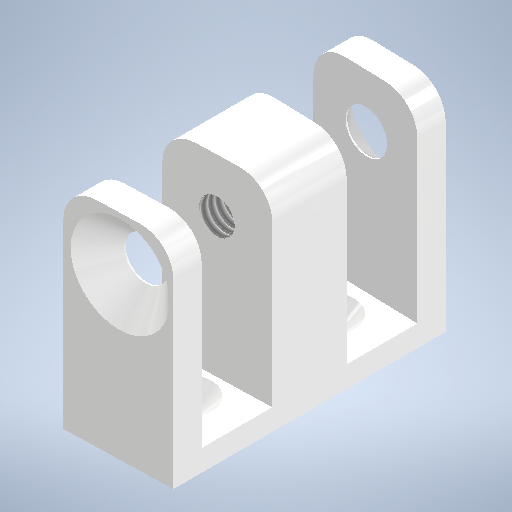
# Autodesk Inventor part: HalterUmlenkrolleDPL
Saved by Autodesk Inventor 2025 (Build 290162010, 162A)
## iProperties
Created: 2024-11-18
Part Number: HalterUmlenkrolleDPL
Material: PC/ABS-Kunststoff, 3DDruck, PLA
Document SubType Name: Modeling
Designer: Admin
Density: 1.1 g/cm^3
Appearance: Glatt - Weiß(2)
Mass: 2.69194 g
Surface Area: 21.9285 cm^2
Volume: 2.44721 cm^3
Author: Admin
Autodesk Inventor part; units mm, degrees
note: some values were not read from the file. Chosen so that the rebuilt part matches the saved one: direction of "Bohrung5"; direction of "Bohrung7".
ref_plane "YZ Plane" through (0, 0, 0) normal (1, 0, 0) x (0, 1, 0)
ref_plane "XZ Plane" through (0, 0, 0) normal (0, 1, 0) x (-1, 0, 0)
ref_plane "XY Plane" through (0, 0, 0) normal (0, 0, 1) x (1, 0, 0)
sketch "Skizze1" plane through (0, 0, 0) normal (0, 0, 1) x (1, 0, 0)
  line L0 (12.8939, 29.9442) -> (2.8939, 30.2214)
  line L1 (2.8939, 30.2214) -> (2.8939, 27.5773)
  line L2 (2.8939, 27.5773) -> (12.8939, 27.3001)
  line L3 (12.8939, 27.3001) -> (12.8939, 29.9442)
  line L4 (12.8939, 7.1427) -> (2.8939, 6.8655)
  line L5 (2.8939, 6.8655) -> (2.8939, 4.2214)
  line L6 (2.8939, 4.2214) -> (12.8939, 4.4985)
  line L7 (12.8939, 4.4985) -> (12.8939, 7.1427)
  line L8 (2.8939, 20.9747) -> (12.8939, 20.6975)
  line L9 (12.8939, 13.7452) -> (2.8939, 13.468)
  line L10 (16.8904, 10.5547) -> (7.8939, 10.3054) construction
  line L11 (16.8904, 23.888) -> (7.8939, 24.1374) construction
  line L12 (16.8904, 10.5547) -> (16.8904, 23.888) construction
  line L13 (2.8939, 20.9747) -> (12.8939, 27.3001) construction
  line L14 (2.8939, 13.468) -> (12.8939, 7.1427) construction
  line L15 (2.8939, 13.468) -> (2.8939, 20.9747)
  line L16 (12.8939, 13.7452) -> (12.8939, 20.6975)
  point P0 (7.8939, 7.0041)
  dimension "d36" = 9
  dimension "d37" = 13.3333
  dimension "d38" = 91.588
  dimension "d39" = 91.588
  dimension "d40" = 10
  dimension "d41" = 6.6
  dimension "d42" = 6.6
  dimension "d43" = 13.8321
  dimension "d58" = 26
  constraints: 34 end point, 6 parallel, 5 collinear, 3 midpoint, 2 vertical, 1 point on line, 1 other
  measures "d36" distance of L10.end L10.start
  measures "d37" distance of L10.start L11.start
  measures "d38" angle of L12 L10
  measures "d39" angle of L12 L11
  measures "d40" distance between parallel lines of L5 L7
  measures "d41" distance between parallel lines of L9 L4
  measures "d42" distance between parallel lines of L2 L8
  measures "d43" distance of L11.end L10.end
  measures "d58" distance of L5.end L0.end
extrude "Extrusion1" add sketch "Skizze1" along normal blind 20
fillet "Rundung1" radius 3 6 edges at (12.8939, 5.8206, 20) (12.8939, 28.6221, 20) (2.8939, 28.8993, 20) (2.8939, 5.5434, 20) (12.8939, 17.2214, 20) (2.8939, 17.2214, 20)
sketch "Skizze4" plane through (2.8939, 22.0416, 0) normal (0, 0, 1) x (1, 0, 0)
  line L0 (9.5, -17.8202) -> (0.5, -17.8202) construction
  line L1 (7, 7.9858) -> (3, 8.0966) construction
  line L2 (5, -11.7363) -> (5, -11.4869) construction
  line L3 (5, 1.8464) -> (5, 2.0958) construction
  dimension "d59" = 13.3333
  constraints: 4 end point, 2 vertical, 1 coincident, 1 collinear
  measures "d59" distance of L2.end L3.start
sketch "Skizze6" plane through (2.8939, 4.2214, 0) normal (0, 0, -1) x (0.9992829, 0.0378646, 0)
  line L0 (10.9668, -25.3257) -> (0.9845, -25.9814) projected
  line L1 (0, 0) -> (10.0033, 0.1017) projected
  line L2 (0.9845, -25.9814) -> (0, 0)
  line L3 (10.9668, -25.3257) -> (10.0033, 0.1017)
  constraints: 4 end point, 1 parallel
extrude "Extrusion3" add sketch "Skizze6" against normal blind 2
hole "Bohrung4" at (7.8939, 10.5547, 0) at (7.8939, 23.888, 0) direction (0, 0, 1) diameter 2 end through all
chamfer "Fasen1" distance 1.5 angle 45 2 edges at (7.8939, 22.888, 2) (7.8939, 9.5547, 2)
sketch "Skizze7" plane through (12.8939, 4.4985, 0) normal (0.0277065, -0.9996161, 0) x (0.9996161, 0.0277065, 0)
  line L0 (-4.8372, 0) -> (-4.8372, 15) construction
  point P0 (-13.0135, 0)
  dimension "d60" = 15
  constraints: 2 end point, 1 coincident, 1 vertical
  measures "d60" distance of L0.start L0.end
hole "Bohrung5" at (8.0585, 4.3645, 15) direction (-0.0277065, 0.9996161, 0) diameter 4 depth 2.6431 countersink diameter 9 countersink angle 90
sketch "Skizze8" plane through (12.8939, 4.4985, 0) normal (0.0277065, -0.9996161, 0) x (0.9996161, 0.0277065, 0)
  circle A0 centre (-4.7839, 15) radius 2.0011 projected
  point P0 (-13.0135, 0)
hole "Bohrung6" at (8.1118, 4.366, 15) direction (-0.0277065, 0.9996161, 0) diameter 3.242 depth 13 tip angle 118 thread size "M4x0.7" class "6H" standard "ANSI Metric M Profile"
sketch "Skizze9" plane through (2.8939, 30.2214, 17) normal (0.0277065, 0.9996161, 0) x (0.9996161, -0.0277065, 0)
  line L0 (5.1666, 17) -> (5.1666, 2) construction
  point P0 (-2.0554, 17)
  dimension "d75" = 15
  constraints: 2 coincident, 2 end point, 1 vertical
  measures "d75" distance of L0.start L0.end
hole "Bohrung7" at (8.0585, 30.0782, 15) direction (-0.0277065, -0.9996161, 0) diameter 4 depth 2.6431 countersink diameter 9 countersink angle 90
sketch "Skizze10" plane through (2.8939, 30.2214, 17) normal (0.0277065, 0.9996161, 0) x (0.9996161, -0.0277065, 0)
  circle A0 centre (5.2233, 2) radius 2.0011 projected
  point P0 (-2.0554, 17)
hole "Bohrung8" at (8.1152, 30.0767, 15) direction (-0.0277065, -0.9996161, 0) diameter 3.242 depth 13 tip angle 118 thread size "M4x0.7" class "6H" standard "ANSI Metric M Profile"
